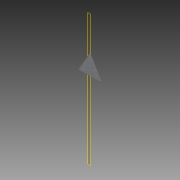
# Autodesk Inventor part: jointplate
Saved by Autodesk Inventor 2014 SP1 (Build 180222100, 222)
## iProperties
Created: 2014-01-06
Part Number: jointplate
Material: Aluminum 6061
Document SubType Name: Modeling
Designer: Arpan
Density: 2.71 g/cm^3
Appearance: Aluminum - Flat
Author: Arpan
Autodesk Inventor part; units mm, degrees
ref_plane "YZ Plane" through (0, 0, 0) normal (1, 0, 0) x (0, 1, 0)
ref_plane "XZ Plane" through (0, 0, 0) normal (0, 1, 0) x (-1, 0, 0)
ref_plane "XY Plane" through (0, 0, 0) normal (0, 0, 1) x (1, 0, 0)
ref_plane "Work Plane1" through (0, 0, 6.9486) normal (0, 0, 1) x (1, 0, 0)
sketch "Sketch1" plane through (0, 0, 6.9486) normal (0, 0, 1) x (1, 0, 0)
  line L0 (-228.6, -575.3768) -> (0, -179.43) projected
  line L1 (254, -575.3768) -> (25.4, -179.43) projected
  line L2 (254, -626.1768) -> (25.4, -230.23) projected
  arc A0 (51.9003, -250.5775) -> (49.8316, -246.9944) centre (50.8, -248.8241) ccw projected
  arc A1 (49.6997, -247.0706) -> (51.7684, -250.6537) centre (50.8, -248.8241) ccw projected
  arc A2 (39.2003, -228.5805) -> (37.1316, -224.9974) centre (38.1, -226.827) ccw projected
  arc A3 (36.9997, -225.0736) -> (39.0684, -228.6567) centre (38.1, -226.827) ccw projected
  arc A4 (12.7762, -217.9687) -> (12.7762, -213.8313) centre (12.7, -215.9) ccw projected
  arc A5 (12.6238, -213.8313) -> (12.6238, -217.9687) centre (12.7, -215.9) ccw projected
  arc A6 (12.6238, -188.4313) -> (12.6238, -192.5687) centre (12.7, -190.5) ccw projected
  arc A7 (12.7762, -192.5687) -> (12.7762, -188.4313) centre (12.7, -190.5) ccw projected
  arc A8 (12.7762, -243.3687) -> (12.7762, -239.2313) centre (12.7, -241.3) ccw projected
  arc A9 (12.6238, -239.2313) -> (12.6238, -243.3687) centre (12.7, -241.3) ccw projected
  arc A10 (-26.3684, -250.6537) -> (-24.2997, -247.0706) centre (-25.4, -248.8241) ccw projected
  arc A11 (-24.4316, -246.9944) -> (-26.5003, -250.5775) centre (-25.4, -248.8241) ccw projected
  arc A12 (-13.6684, -228.6567) -> (-11.5997, -225.0736) centre (-12.7, -226.827) ccw projected
  arc A13 (-11.7316, -224.9974) -> (-13.8003, -228.5805) centre (-12.7, -226.827) ccw projected
  line L3 (12.7, -241.3) -> (12.7, -266.7)
  line L4 (12.7, -266.7) -> (-50.3854, -266.7)
  line L5 (12.7, -266.7) -> (75.7854, -266.7)
  line L6 (75.7854, -266.7) -> (12.7, -157.4329)
  line L7 (-50.3854, -266.7) -> (12.7, -157.4329)
  circle A14 centre (12.7, -190.5) radius 2.0701
  circle A15 centre (12.7, -215.9) radius 2.0701
  circle A16 centre (12.7, -241.3) radius 2.0701
  circle A17 centre (-25.4, -248.8241) radius 2.0701
  circle A18 centre (-12.7, -226.827) radius 2.0701
  circle A19 centre (50.8, -248.8241) radius 2.0701
  circle A20 centre (38.1, -226.827) radius 2.0701
  point P0 (0, 0)
  dimension "d0" = 25.4
  constraints: 10 end point, 7 centre point, 7 coincident, 5 concentric, 2 collinear, 2 point on line, 1 parallel, 1 perpendicular, 1 vertical
  measures "d0" distance of L3.start L3.end
extrude "Extrusion1" add sketch "Sketch1" along normal blind 3.175
fillet "Fillet1" radius 3.175 3 edges at (12.7, -157.4329, 8.5361) (-50.3854, -266.7, 8.5361) (75.7854, -266.7, 8.5361)
body "Solid1"
